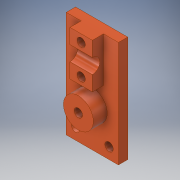
# Autodesk Inventor part: X-axis Idler
Saved by Autodesk Inventor 2018 (Build 220112000, 112)
## iProperties
Created: 2013-10-27
Part Number: X-axis Idler
Material: ABS Plastic
Document SubType Name: Modeling
Designer: Gabriel Smolnycki
Mass: 10.819 g
Surface Area: 53.2558 cm^2
Volume: 10.2066 cm^3
Density: 1.06 g/cm^3
Appearance: Smooth - Light Orange
Author: Gabriel Smolnycki
Sending System: SolidWorks 2017
Last Author: Gabriel Smolnycki
Last Saved: 2017-09-14
Autodesk Inventor part; units mm, degrees
ref_plane "YZ Plane" through (0, 0, 0) normal (1, 0, 0) x (0, 1, 0)
ref_plane "XZ Plane" through (0, 0, 0) normal (0, 1, 0) x (-1, 0, 0)
ref_plane "XY Plane" through (0, 0, 0) normal (0, 0, 1) x (1, 0, 0)
sketch "Sketch1" plane through (0, 0, 0) normal (0, 0, 1) x (1, 0, 0)
  line L0 (-14, 0) -> (-14, -57)
  line L1 (14, -57) -> (14, 0)
  line L2 (14, 0) -> (-14, 0)
  line L3 (-14, -57) -> (14, -57)
  constraints: 8 end point, 2 horizontal, 2 vertical
extrude "Extrusion3" add sketch "Sketch1" along normal blind 5
sketch "Sketch2" plane through (0, 0, 5) normal (0, 0, 1) x (1, 0, 0)
  circle A0 centre (0, -36) radius 8
  constraints: 1 centre point
extrude "Extrusion2" add sketch "Sketch2" along normal blind 7.5
sketch "Sketch3" plane through (0, 0, 0) normal (0, 1, 0) x (-1, 0, 0)
  line L0 (6, 5) -> (-6, 5)
  line L1 (6, 11) -> (-6, 11)
  line L2 (6, 11) -> (6, 5)
  line L3 (-6, 11) -> (-6, 5)
  constraints: 8 end point, 2 horizontal, 2 vertical
extrude "Extrusion1" add sketch "Sketch3" against normal blind 24
hole "Hole5" at (0, -36, 0) direction (0, 0, 1) diameter 4.5 depth 12.5 tip angle 118
hole "Hole4" at (9, -51, 0) direction (0, 0, 1) diameter 4.5 depth 5 tip angle 118
sketch "Sketch6" plane through (0, 0, 0) normal (0, 0, 1) x (1, 0, 0)
  point P0 (-9, -51)
hole "Hole3" at (-9, -51, 0) direction (0, 0, 1) diameter 4.5 depth 5 tip angle 118
sketch "Sketch5" plane through (0, 0, 0) normal (0, 0, 1) x (1, 0, 0)
  point P0 (9, -51)
hole "Hole2" at (0, -20, 0) direction (0, 0, 1) diameter 4.5 depth 11 tip angle 118
sketch "Sketch4" plane through (0, 0, 0) normal (0, 0, 1) x (1, 0, 0)
  point P0 (0, -36)
hole "Hole1" at (0, -4, 0) direction (0, 0, 1) diameter 4.5 depth 11 tip angle 118
sketch "Sketch9" plane through (-6, 0, 11) normal (0, 0, 1) x (1, 0, 0)
  line L0 (0, -8) -> (12, -8)
  line L1 (0, -8) -> (0, -12)
  line L2 (12, -8) -> (12, -12)
  line L3 (0, -12) -> (12, -12)
  line L4 (0, -12) -> (10, -12)
  constraints: 10 end point, 3 horizontal, 2 vertical
revolve "Revolution1" cut sketch "Sketch9" angle 180 about axis through (-6, -12, 11) along (-1, 0, 0)
sketch "Sketch7" plane through (0, 0, 0) normal (0, 0, 1) x (1, 0, 0)
  point P0 (0, -20)
sketch "Sketch8" plane through (0, 0, 0) normal (0, 0, 1) x (1, 0, 0)
  point P0 (0, -4)
body "Solid3"
